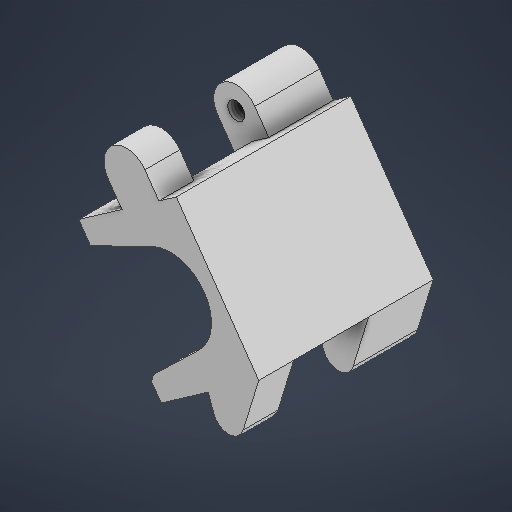
# Autodesk Inventor part: F3_Rough_Rear_Caliper_V2
Saved by Autodesk Inventor 2026.1 (Build 301233000, 233)
## iProperties
Created: 2026-09-12
Part Number: F3_Rough_Rear_Caliper_V2
Material: Generic
Document SubType Name: Modeling
Designer: share
Density: 1 g/cm^3
Appearance: Default
Author: share
Autodesk Inventor part; units mm, degrees
ref_plane "YZ Plane" through (0, 0, 0) normal (1, 0, 0) x (0, 1, 0)
ref_plane "XZ Plane" through (0, 0, 0) normal (0, 1, 0) x (-1, 0, 0)
sketch "Sketch1" plane through (0, 0, 0) normal (0, 0, 1) x (1, 0, 0)
  circle A0 centre (20, 109) radius 11
  circle A1 centre (20, 20) radius 13
  line L0 (20, 109) -> (20, 20) construction
  line L1 (0, 144) -> (0, -24) construction
  line L2 (-16.8865, 0) -> (101.3193, 0) construction
  circle A2 centre (30, 60) radius 24
  line L3 (23.5359, 84.7724) -> (16.2342, 79.6596)
  line L4 (10.9893, 102.6907) -> (23.5359, 84.7724)
  line L5 (30, 60) -> (20, 20) construction
  line L6 (15.0071, 41.2593) -> (12.3132, 30.484)
  line L7 (34.4099, 36.4086) -> (31.7161, 25.6333)
  line L8 (29.0107, 115.3093) -> (35.8214, 105.5826)
  line L9 (35.8214, 105.5826) -> (44.2824, 111.507)
  line L10 (44.2824, 111.507) -> (84.4327, 54.1663)
  line L11 (84.4327, 54.1663) -> (38.1631, 37.4309)
  circle A3 centre (69.6897, 31.6354) radius 7.5
  line L12 (84.4327, 54.1663) -> (76.861, 29.4394)
  line L13 (62.6369, 29.0844) -> (57.1359, 44.2933)
  point P0 (0, 0)
  dimension "d0" = 89
  dimension "d2" = 48
  dimension "d3" = 20
  dimension "d4" = 20
  dimension "d5" = 26
  dimension "d6" = 22
  dimension "d7" = 40
  dimension "d8" = 10
  dimension "d9" = 35
  dimension "d10" = 20
  dimension "d11" = 10
  dimension "d13" = 10.3289
  dimension "d14" = 70
  dimension "d15" = 25
  dimension "d17" = 80
  dimension "d18" = 15
  constraints: 24 end point, 10 point on circle, 6 tangent, 5 parallel, 4 centre point, 3 perpendicular, 1 point on line, 1 other
  measures "d0" distance of L0.start L0.end
  measures "d2" diameter of A2
  measures "d3" distance from line of L0.end L1
  measures "d4" distance from line of L2 L0.end
  measures "d5" diameter of A1
  measures "d6" diameter of A0
  measures "d7" vertical distance of L0.end L5.start
  measures "d8" distance from line of L5.start L0
  measures "d9" angle of L3 L2
  measures "d10" distance between parallel lines of L6 L7
  measures "d11" distance between parallel lines of L3 L9
  measures "d13" distance between parallel lines of L10 L8
  measures "d14" distance of L9.end L10.end
  measures "d15" distance from line of L10 A3.centre
  measures "d17" distance from line of A3.centre L9
  measures "d18" diameter of A3
extrude "Extrusion1" add sketch "Sketch1" against normal blind 38
ref_plane "Work Plane1" through (0, 0, 30) normal (0, 0, 1) x (1, 0, 0)
sketch "Sketch2" plane through (0, 0, 30) normal (0, 0, 1) x (1, 0, 0)
  line L0 (10.9893, 102.6907) -> (23.5359, 84.7724) projected
  line L1 (23.5359, 84.7724) -> (16.2342, 79.6596) projected
  arc A0 (16.2342, 79.6596) -> (15.0071, 41.2593) centre (30, 60) ccw projected
  line L2 (15.0071, 41.2593) -> (12.3132, 30.484) projected
  arc A1 (12.3132, 30.484) -> (31.7161, 25.6333) centre (20, 20) ccw projected
  line L3 (31.7161, 25.6333) -> (34.4099, 36.4086) projected
  arc A2 (34.4099, 36.4086) -> (38.1631, 37.4309) centre (30, 60) ccw projected
  line L4 (38.1631, 37.4309) -> (57.1359, 44.2933) projected
  line L5 (57.1359, 44.2933) -> (62.6369, 29.0844) projected
  arc A3 (62.6369, 29.0844) -> (76.861, 29.4394) centre (69.6897, 31.6354) ccw projected
  line L6 (76.861, 29.4394) -> (84.4327, 54.1663) projected
  line L7 (84.4327, 54.1663) -> (44.2824, 111.507) projected
  arc A4 (29.0107, 115.3093) -> (10.9893, 102.6907) centre (20, 109) ccw projected
  line L8 (84.4327, 54.1663) -> (36.9219, 20.8989)
  line L9 (44.2824, 111.507) -> (-3.2284, 78.2395)
  line L10 (35.8214, 105.5826) -> (29.0107, 115.3093) projected
  line L11 (-3.2284, 78.2395) -> (2.5073, 70.048)
  line L12 (36.9219, 20.8989) -> (31.1862, 29.0904)
  line L13 (2.5073, 70.048) -> (31.1862, 29.0904) construction
  circle A5 centre (41.4213, 66.7765) radius 20
  line L14 (41.4213, 66.7765) -> (16.8468, 49.5692) construction
  line L15 (2.5073, 70.048) -> (32.6535, 84.7522)
  line L16 (31.1862, 29.0904) -> (55.3141, 52.3894)
  point P0 (0, 0)
  point P1 (17.8001, 92.9639)
  point P2 (33.0241, 30.8652)
  point P3 (32.2136, 27.6232)
  point P4 (59.8027, 36.9202)
  dimension "d23" = 58
  dimension "d27" = 10
  dimension "d28" = 30
  dimension "d29" = 40
  constraints: 16 end point, 6 centre point, 5 perpendicular, 2 equal length, 2 point on circle, 2 tangent, 1 collinear, 1 midpoint
  measures "d23" distance of L7.end L9.end
  measures "d27" distance of L9.end L11.end
  measures "d28" distance of L14.start L14.end
  measures "d29" diameter of A5
extrude "Extrusion2" add sketch "Sketch2" along normal blind 17 contours A4 L10 L9 L0 | L9 L7 L8 L5 L4 L16 A5 L15 A0 L1 L0 | L0 L1 A0 L15 L11 L9 | L6 A3 L5 L8 | L8 L12 L3 L16 L4 L5
sketch "Sketch3" plane through (0, 0, 30) normal (0, 0, -1) x (-1, 0, 0)
  line L0 (-10.9893, 102.6907) -> (-17.8001, 92.9639) projected
  arc A0 (-10.9893, 102.6907) -> (-29.0107, 115.3093) centre (-20, 109) ccw projected
  line L1 (-35.8214, 105.5826) -> (-29.0107, 115.3093) projected
  line L2 (-44.2824, 111.507) -> (-35.8214, 105.5826) projected
  line L3 (-84.4327, 54.1663) -> (-44.2824, 111.507) projected
  line L4 (-76.861, 29.4394) -> (-84.4327, 54.1663) projected
  arc A1 (-76.861, 29.4394) -> (-62.6369, 29.0844) centre (-69.6897, 31.6354) ccw projected
  line L5 (-59.8027, 36.9202) -> (-62.6369, 29.0844) projected
  line L6 (-36.9219, 20.8989) -> (-59.8027, 36.9202) projected
  line L7 (-32.2136, 27.6232) -> (-36.9219, 20.8989) projected
  line L8 (-33.0241, 30.8652) -> (-32.2136, 27.6232) projected
  line L9 (-55.3141, 52.3894) -> (-33.0241, 30.8652) projected
  arc A2 (-32.6535, 84.7522) -> (-55.3141, 52.3894) centre (-41.4213, 66.7765) ccw projected
  line L10 (-2.5073, 70.048) -> (-32.6535, 84.7522) projected
  line L11 (3.2284, 78.2395) -> (-2.5073, 70.048) projected
  line L12 (-17.8001, 92.9639) -> (3.2284, 78.2395) projected
  line L13 (-59.8027, 36.9202) -> (-84.4327, 54.1663)
  line L14 (-35.8214, 105.5826) -> (-17.8001, 92.9639)
  line L15 (-27.8994, 100.0354) -> (-37.4607, 86.3804)
  line L16 (-84.4327, 54.1663) -> (-44.2824, 111.507) projected
  line L17 (-68.0497, 42.6948) -> (-58.4884, 56.3498)
  line L18 (-32.493, 93.475) -> (-48.8761, 104.9465) construction
  line L19 (-63.269, 49.5223) -> (-79.6521, 60.9938) construction
  point P0 (0, 0)
  dimension "d52" = 20
  constraints: 12 end point, 5 point on line, 3 perpendicular, 2 parallel, 2 point on circle, 1 midpoint
  measures "d52" distance between parallel lines of L17 L3
extrude "Extrusion3" add sketch "Sketch3" along normal up to surface (30 mm away) contours L15 A2 L17 L13 L3 L2 L14
sketch "Sketch4" plane through (0, 0, 0) normal (0, 0, 1) x (1, 0, 0)
  arc A0 (29.0107, 115.3093) -> (10.9893, 102.6907) centre (20, 109) ccw projected
  point P0 (0, 0)
  constraints: 1 coincident
hole "Hole1" at (20, 109, 0) direction (0, 0, -1) diameter 8.376 end through all thread size "M10x1.5" class "6H" standard "ANSI Metric M Profile"
sketch "Sketch5" plane through (0, 0, 0) normal (0, 0, 1) x (1, 0, 0)
  arc A0 (12.3132, 30.484) -> (31.7161, 25.6333) centre (20, 20) ccw projected
  point P0 (0, 0)
  constraints: 1 coincident
hole "Hole2" at (20, 20, 0) direction (0, 0, -1) diameter 6 end through all
sketch "Sketch6" plane through (0, 0, 0) normal (0, 0, 1) x (1, 0, 0)
  circle A0 centre (20, 20) radius 3 projected
  circle A1 centre (20, 109) radius 4.188 projected
  arc A2 (58.4884, 56.3498) -> (37.4607, 86.3804) centre (41.4213, 66.7765) ccw projected
  line L0 (27.8994, 100.0354) -> (35.8214, 105.5826) projected
  line L1 (35.8214, 105.5826) -> (29.0107, 115.3093) projected
  arc A3 (29.0107, 115.3093) -> (10.9893, 102.6907) centre (20, 109) ccw projected
  line L2 (10.9893, 102.6907) -> (23.5359, 84.7724) projected
  arc A4 (16.2342, 79.6596) -> (15.0071, 41.2593) centre (30, 60) ccw projected
  line L3 (15.0071, 41.2593) -> (12.3132, 30.484) projected
  arc A5 (12.3132, 30.484) -> (31.7161, 25.6333) centre (20, 20) ccw projected
  line L4 (31.7161, 25.6333) -> (34.4099, 36.4086) projected
  arc A6 (34.4099, 36.4086) -> (38.1631, 37.4309) centre (30, 60) ccw projected
  line L5 (38.1631, 37.4309) -> (57.1359, 44.2933) projected
  line L6 (34.4099, 36.4086) -> (15.0071, 41.2593)
  line L7 (84.4327, 54.1663) -> (68.0497, 42.6948) projected
  line L8 (68.0497, 42.6948) -> (58.4884, 56.3498) projected
  line L9 (37.4607, 86.3804) -> (27.8994, 100.0354) projected
  line L10 (23.5359, 84.7724) -> (16.2342, 79.6596) projected
  line L11 (57.1359, 44.2933) -> (62.6369, 29.0844) projected
  arc A7 (62.6369, 29.0844) -> (76.861, 29.4394) centre (69.6897, 31.6354) ccw projected
  line L12 (76.861, 29.4394) -> (84.4327, 54.1663) projected
  point P0 (0, 0)
  constraints: 2 end point
extrude "Extrusion4" cut sketch "Sketch6" against normal blind 10 contours L4 A5 L3 L6
sketch "Sketch7" plane through (0, 0, 0) normal (0, 0, 1) x (1, 0, 0)
  line L0 (15.0071, 41.2593) -> (34.4099, 36.4086) projected
  arc A0 (34.4099, 36.4086) -> (38.1631, 37.4309) centre (30, 60) ccw projected
  line L1 (38.1631, 37.4309) -> (57.1359, 44.2933) projected
  arc A1 (58.4884, 56.3498) -> (37.4607, 86.3804) centre (41.4213, 66.7765) ccw projected
  line L2 (27.8994, 100.0354) -> (35.8214, 105.5826) projected
  line L3 (35.8214, 105.5826) -> (29.0107, 115.3093) projected
  arc A2 (29.0107, 115.3093) -> (10.9893, 102.6907) centre (20, 109) ccw projected
  line L4 (10.9893, 102.6907) -> (23.5359, 84.7724) projected
  arc A3 (16.2342, 79.6596) -> (15.0071, 41.2593) centre (30, 60) ccw projected
  circle A4 centre (20, 109) radius 4.188 projected
  line L5 (19.6524, 94.2609) -> (17.2626, 93.7315)
  line L6 (57.1359, 44.2933) -> (62.6369, 29.0844) projected
  arc A5 (62.6369, 29.0844) -> (76.861, 29.4394) centre (69.6897, 31.6354) ccw projected
  line L7 (76.861, 29.4394) -> (84.4327, 54.1663) projected
  line L8 (84.4327, 54.1663) -> (68.0497, 42.6948) projected
  line L9 (68.0497, 42.6948) -> (58.4884, 56.3498) projected
  line L10 (37.4607, 86.3804) -> (27.8994, 100.0354) projected
  line L11 (23.5359, 84.7724) -> (16.2342, 79.6596) projected
  point P0 (0, 0)
  constraints: 2 end point, 1 midpoint
extrude "Extrusion5" cut sketch "Sketch7" against normal blind 6.5
body "Solid1"
